gantry_frame_bumper (Autodesk Fusion 360 design; units mm, degrees)
Autodesk Fusion 360 part; units mm, degrees
sketch "Sketch1" plane through (0, 0, 0) normal (0, 0, 1) x (1, 0, 0)
  line L0 (20, -10) -> (-20, -10)
  line L1 (-20, -10) -> (-20, 10)
  line L2 (-20, 10) -> (20, 10)
  line L3 (20, 10) -> (20, -10)
  line L4 (20, -10) -> (-20, 10) construction
  line L5 (-20, -10) -> (20, 10) construction
  line L6 (-20, 0) -> (20, 0) construction
  circle A0 centre (-10, 0) radius 1.7
  circle A1 centre (-10, 0) radius 3
  line L7 (0, 10) -> (0, -10) construction
  circle A2 centre (10, 0) radius 1.7
  circle A3 centre (10, 0) radius 3
  line L8 (-6.1906, 3.4245) -> (-13.346, 7.0022)
  line L9 (-13.346, 7.0022) -> (-12.8094, 8.0755)
  line L10 (-12.8094, 8.0755) -> (-5.654, 4.4978)
  line L11 (-5.654, 4.4978) -> (-6.1906, 3.4245)
  line L12 (-6.1906, 3.4245) -> (-12.8094, 8.0755) construction
  line L13 (-13.346, 7.0022) -> (-5.654, 4.4978) construction
  line L14 (6.1906, 3.4245) -> (13.346, 7.0022)
  line L15 (13.346, 7.0022) -> (12.8094, 8.0755)
  line L16 (12.8094, 8.0755) -> (5.654, 4.4978)
  line L17 (5.654, 4.4978) -> (6.1906, 3.4245)
  line L18 (-13.0094, 7.6755) -> (-12.0094, 7.6755)
  line L19 (13.0094, 7.6755) -> (12.0094, 7.6755)
  point P0 (-9.5, 5.75)
  dimension "d1" = 40
  dimension "d2" = 20
  dimension "d3" = 3.4
  dimension "d4" = 6
  dimension "d5" = 10
  dimension "d17" = 8
  dimension "d18" = 1.2
  dimension "d19" = 9.5
  dimension "d20" = 4.25
  dimension "d24" = 0.4
  constraint horizontal L0
  constraint perpendicular L0 L1
  constraint parallel L0 L2
  constraint parallel L1 L3
  constraint coincident L4 origin
  constraint coincident L5 origin
  constraint midpoint L1 L6.start
  constraint midpoint L3 L6.end
  constraint coincident L6 A0.centre
  constraint concentric A0 A1
  constraint midpoint L2 L7.start
  constraint midpoint L0 L7.end
  constraint symmetric A0 L7 A2
  constraint symmetric A1 L7 A3
  constraint perpendicular L8 L9
  constraint parallel L8 L10
  constraint parallel L9 L11
  constraint coincident L12 P0
  constraint coincident L13 P0
  constraint parallel L4 L10
  constraint symmetric L7 L8.start L14.start
  constraint symmetric L7 L8.end L14.end
  constraint symmetric L7 L9.end L15.end
  constraint symmetric L7 L10.end L16.end
  constraint coincident L10 L18.end
  constraint horizontal L18
  constraint coincident L9 L18.start
  constraint symmetric L7 L18.start L19.start
  constraint symmetric L7 L18.end L19.end
  measures "d1" distance of L1.end L2.end
  measures "d2" distance of L0.end L1.end
  measures "d3" diameter of A0
  measures "d4" diameter of A1
  measures "d5" distance of L6.start A0.centre
  measures "d17" distance of L9.end L10.end
  measures "d18" distance of L8.end L9.end
  measures "d19" distance of L7 P0
  measures "d20" vertical distance of L7.start P0
  measures "d24" distance of L9.end L18
extrude "Extrude1" add sketch "Sketch1" along normal blind 18 contours L0 L1 L2 L3 | A1 | A3 | L8 L9 L10 L11 L18 | L9 L10 L18 | L14 L15 L16 L17 L19 | L15 L16 L19
extrude "Extrude2" cut sketch "Sketch1" against normal blind 3 from surface at 18 contours A1 | A3
fillet "Fillet1" radius 3 4 edges at (-20, 10, 9) (-20, -10, 9) (20, -10, 9) (20, 10, 9)
chamfer "Chamfer1" distance 1 angle 45 8 edges at (0, 10, 18) (-19.1213, 9.1213, 18) (-20, 0, 18) (-19.1213, -9.1213, 18) (0, -10, 18) (19.1213, -9.1213, 18) (20, 0, 18) (19.1213, 9.1213, 18)
chamfer "Chamfer2" distance 0.4 angle 45 10 edges at (7.203, 1.0848, 18) (-12.797, 1.0848, 18) (0, -10, 0) (-19.1213, -9.1213, 0) (-20, 0, 0) (-19.1213, 9.1213, 0) (0, 10, 0) (19.1213, 9.1213, 0) (20, 0, 0) (19.1213, -9.1213, 0)
chamfer "Chamfer3" distance 0.2 angle 45 2 edges at (-11.585, -0.6147, 15) (8.415, -0.6147, 15)
chamfer "Chamfer4" distance 0.4 angle 45 2 edges at (-11.585, 0.6147, 0) (8.415, 0.6147, 0)
extrude "Extrude3" cut sketch "Sketch1" against normal blind 0.8 from surface at 18 contours L8 L9 L10 L11 L18 | L14 L15 L16 L17 L19
